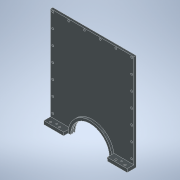
# Autodesk Inventor part: Крышка стенки картера верх
Saved by Autodesk Inventor 2021 (Build 250183000, 183)
## iProperties
Created: 2020-12-06
Part Number: Крышка стенки картера верх
Material: Чугун, серый
Document SubType Name: Modeling
Designer: Тимоха
Density: 7.15 g/cm^3
Appearance: Чугун серый
Mass: 11250.7 g
Surface Area: 3356.36 cm^2
Volume: 1573.52 cm^3
Author: Тимоха
Autodesk Inventor part; units mm, degrees
ref_plane "YZ Plane" through (0, 0, 0) normal (1, 0, 0) x (0, 1, 0)
ref_plane "XZ Plane" through (0, 0, 0) normal (0, 1, 0) x (-1, 0, 0)
ref_plane "РабПлоскость1" through (0, 0, 0) normal (0, 0, 1) x (1, 0, 0)
sketch "Эскиз1" plane through (0, 0, 0) normal (0, 0, 1) x (1, 0, 0)
  line L0 (185, -75) -> (185, 325) projected
  line L1 (165, 340) -> (165, -75) projected
  arc A0 (-165, -75) -> (165, -75) centre (0, -75) ccw projected
  line L2 (-165, -75) -> (-165, 340) projected
  line L3 (-185, 325) -> (-185, -75) projected
  arc A1 (-185, -75) -> (185, -75) centre (0, -75) ccw projected
  line L4 (185, -75) -> (97.5, -75) projected
  line L5 (-97.5, -75) -> (-185, -75) projected
  line L6 (-185, -75) -> (185, -75)
  line L7 (-185, 340) -> (-185, 355)
  line L8 (-185, 355) -> (185, 355)
  line L9 (185, 355) -> (185, 338)
  line L10 (185, 325) -> (230, 325) projected
  line L11 (230, 325) -> (230, 340) projected
  line L12 (230, 340) -> (165, 340) projected
  line L13 (-165, 340) -> (-230, 340) projected
  line L14 (-230, 340) -> (-230, 325) projected
  line L15 (-230, 325) -> (-185, 325) projected
  line L16 (-185, 340) -> (-185, 325)
  line L17 (185, 340) -> (185, 325)
  point P0 (0, 0)
  point P1 (-97.5, -75)
  point P2 (165, -75)
  point P3 (-165, -75)
  point P4 (-185, -75)
  point P5 (-165, -75)
  point P6 (185, -75)
  dimension "d0" = 15
  dimension "d1" = 370
  constraints: 13 end point, 2 collinear, 1 perpendicular, 1 point on line, 1 vertical
  measures "d0" distance of L7.start L7.end
  measures "d1" distance of L7.end L8.end
extrude "Выдавливание1" add sketch "Эскиз1" along normal blind 10 contours L4 L1 L12 L9 L17 L0 | L3 L16 L13 L2 L5 | L4 L6 L5 L2 L13 L7 L8 L9 L12 L1
sketch "Эскиз2" plane through (0, 0, 10) normal (0, 0, 1) x (1, 0, 0)
  arc A0 (-96.3392, -90) -> (96.3392, -90) centre (0, -75) ccw projected
  arc A1 (-86, -75) -> (86, -75) centre (0, -75) ccw projected
  circle A2 centre (0, -75) radius 86
  line L0 (-185, -75) -> (185, -75) projected
  line L1 (-97.3373, -75) -> (97.3373, -75)
  circle A3 centre (0, -75) radius 97.3373
  point P0 (0, 0)
  point P1 (86, -75)
  point P2 (-165, -75)
  point P3 (165, -75)
  constraints: 2 end point, 2 point on line, 1 centre point, 1 coincident, 1 concentric, 3 other
extrude "Выдавливание2" add sketch "Эскиз2" along normal blind 10 contours L0 A3 A2
sketch "Эскиз3" plane through (0, 0, 10) normal (0, 0, 1) x (1, 0, 0)
  arc A0 (86, -75) -> (-86, -75) centre (0, -75) ccw projected
  line L0 (185, 355) -> (-185, 355) projected
  line L1 (-185, 355) -> (-185, -75) projected
  arc A1 (97.3373, -75) -> (-97.3373, -75) centre (0, -75) ccw projected
  line L2 (-86, -75) -> (86, -75) projected
  line L3 (97.3373, -75) -> (185, -75) projected
  line L4 (185, -75) -> (185, 355) projected
  line L5 (-185, -75) -> (-97.3373, -75) projected
  point P0 (0, 0)
extrude "Выдавливание3" cut sketch "Эскиз3" against normal through all contours L2 A0
sketch "Эскиз8" plane through (0, 0, 10) normal (0, 0, 1) x (1, 0, 0)
  line L0 (-185, 355) -> (-185, -75) projected
  line L1 (-185, 355) -> (-175, 355)
  line L2 (185, 355) -> (-185, 355) projected
  line L3 (-175, 355) -> (-175, 348)
  point P0 (0, 0)
  constraints: 4 end point, 1 point on line, 1 vertical
hole "Отверстие1" at (-175, 348, 10) direction (0, 0, -1) diameter 9 end through all
pattern_linear "Прямоуг.массив1" count 7 spacing 65 along (0, -1, 0) of "Отверстие1"
mirror "Зеркальное отражение1" about plane through (0, 0, 0) normal (1, 0, 0) of "Отверстие1", "Прямоуг.массив1"
pattern_linear "Прямоуг.массив2" count 5 spacing 70 along (1, 0, 0) of "Отверстие1"
sketch "Эскиз9" plane through (0, 0, 10) normal (0, 0, 1) x (1, 0, 0)
  circle A0 centre (105, 348) radius 4.5 projected
  circle A1 centre (35, 348) radius 4.5 projected
  circle A2 centre (-35, 348) radius 4.5 projected
  circle A3 centre (-105, 348) radius 4.5 projected
  circle A4 centre (175, -42) radius 4.5 projected
  circle A5 centre (175, 23) radius 4.5 projected
  circle A6 centre (175, 88) radius 4.5 projected
  circle A7 centre (175, 153) radius 4.5 projected
  circle A8 centre (175, 218) radius 4.5 projected
  circle A9 centre (175, 283) radius 4.5 projected
  circle A10 centre (175, 348) radius 4.5 projected
  circle A11 centre (-175, -42) radius 4.5 projected
  circle A12 centre (-175, 23) radius 4.5 projected
  circle A13 centre (-175, 88) radius 4.5 projected
  circle A14 centre (-175, 153) radius 4.5 projected
  circle A15 centre (-175, 218) radius 4.5 projected
  circle A16 centre (-175, 283) radius 4.5 projected
  circle A17 centre (-175, 348) radius 4.5 projected
  arc A18 (97.3373, -75) -> (-97.3373, -75) centre (0, -75) ccw projected
  line L0 (97.3373, -75) -> (185, -75) projected
  line L1 (185, -75) -> (185, 355) projected
  line L2 (185, 355) -> (-185, 355) projected
  line L3 (-185, 355) -> (-185, -75) projected
  line L4 (-185, -75) -> (-97.3373, -75) projected
  line L5 (-185, -75) -> (-185, -60)
  line L6 (-185, 355) -> (-185, -75) projected
  line L7 (-185, -60) -> (-96.1746, -60)
  arc A19 (97.3373, -75) -> (-97.3373, -75) centre (0, -75) ccw projected
  line L8 (185, -75) -> (185, 355) projected
  line L9 (185, -75) -> (185, -60)
  line L10 (185, -60) -> (96.1746, -60)
  point P0 (0, 0)
  point P1 (-96.1746, -60)
  dimension "d31" = 15
  dimension "d32" = 15
  constraints: 8 end point, 3 point on line, 2 point on circle, 1 perpendicular
  measures "d31" distance of L3.end L5.end
  measures "d32" distance of L0.end L9.end
extrude "Выдавливание7" add sketch "Эскиз9" along normal blind 30 contours A18 L10 L1 L0 | A18 L4 L3 L7
sketch "Эскиз10" plane through (-185, -60, 10) normal (0, 1, 0) x (1, 0, 0)
  circle A0 centre (20, -20) radius 4 projected
  circle A1 centre (41, -14) radius 3 projected
  circle A2 centre (60, -20) radius 4 projected
  circle A3 centre (310, -20) radius 4 projected
  circle A4 centre (329, -14) radius 3 projected
  circle A5 centre (350, -20) radius 4 projected
  point P0 (185, 10)
extrude "Выдавливание8" cut sketch "Эскиз10" against normal blind 30
sketch "Эскиз11" plane through (86, -75, 0) normal (0, -1, 0) x (1, 0, 0)
  line L0 (7, 17) -> (0, 17)
  line L1 (7, 12) -> (7, 17)
  line L2 (0, 12) -> (7, 12)
  line L3 (7, 9) -> (0, 9)
  line L4 (7, 3) -> (7, 9)
  line L5 (0, 3) -> (7, 3)
  line L6 (-86, 0) -> (-86, 42)
  line L7 (0, 17) -> (0, 3)
  constraints: 16 end point, 4 horizontal, 3 vertical, 1 perpendicular, 8 other
revolve "Вращение2" cut sketch "Эскиз11" angle 360 about axis through (0, -75, 0) along (0, 0, 1)
